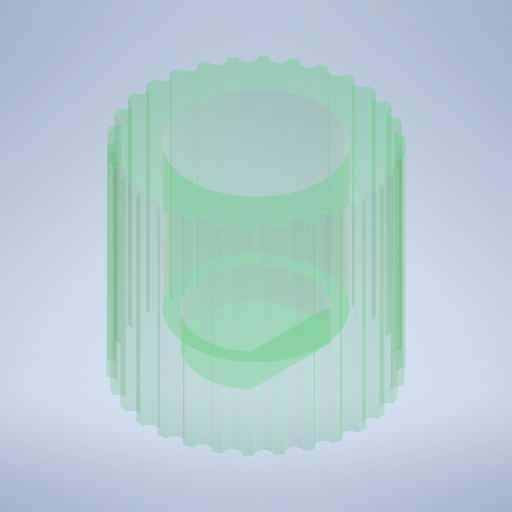
# Autodesk Inventor part: Knob Rotory Encoder
Saved by Autodesk Inventor 2024 (Build 280153000, 153)
## iProperties
Created: 2024-09-25
Part Number: Knob Rotory Encoder
Material: Generic
Document SubType Name: Modeling
Designer: Emil
Density: 1 g/cm^3
Appearance: Clear - Green 1
Author: Emil
Autodesk Inventor part; units mm, degrees
ref_plane "YZ Plane" through (0, 0, 0) normal (1, 0, 0) x (0, 1, 0)
ref_plane "XZ Plane" through (0, 0, 0) normal (0, 1, 0) x (-1, 0, 0)
ref_plane "XY Plane" through (0, 0, 0) normal (0, 0, 1) x (1, 0, 0)
sketch "Sketch1" plane through (0, 0, 0) normal (0, 1, 0) x (-1, 0, 0)
  circle A0 centre (0, 0) radius 6
  dimension "d0" = 12
  constraints: 1 centre point, 1 coincident
  measures "d0" diameter of A0
extrude "Extrusion1" add sketch "Sketch1" along normal blind 3
sketch "Sketch2" plane through (0, 3, 0) normal (0, 1, 0) x (1, 0, 0)
  circle A0 centre (0, 0) radius 3.025
  line L0 (1.975, -3) -> (1.975, 3)
  line L1 (-3.025, 0) -> (1.975, 0)
  point P0 (1.975, 2.2913)
  point P1 (1.975, -2.2913)
  dimension "d3" = 6.05
  dimension "d4" = 5
  constraints: 4 end point, 1 coincident, 1 midpoint, 1 vertical, 3 other
  measures "d4" distance of L1.start L1.end
extrude "Extrusion2" cut sketch "Sketch2" against normal blind 1.86 contours L0 L1 A0 | A0 L1 L0
sketch "Sketch4" plane through (0, 3, 0) normal (0, 1, 0) x (1, 0, 0)
  circle A0 centre (0, 0) radius 3.75
  circle A1 centre (0, 0) radius 6
  dimension "d15" = 7.5
  dimension "d16" = 12
  constraints: 2 centre point, 2 coincident
  measures "d15" diameter of A0
  measures "d16" diameter of A1
extrude "Extrusion4" add sketch "Sketch4" along normal blind 8.14
sketch "Sketch5" plane through (0, 0, 0) normal (0, -1, 0) x (1, 0, 0)
  circle A0 centre (0, 0) radius 6 projected
  circle A1 centre (0, 6) radius 0.4
  dimension "d17" = 0.8
  constraints: 1 centre point, 1 vertical alignment, 1 other
  measures "d17" diameter of A1
extrude "Extrusion5" cut sketch "Sketch5" against normal through all contours A1 A0 | A0 A1 picked at (-0.0157, 5.8666) picked at (0.014, 6.1316)
pattern_circular "Circular Pattern2" count 30 over 360 about axis through (0, 0, 0) along (0, 1, 0) of "Extrusion5"
body "Solid1"
